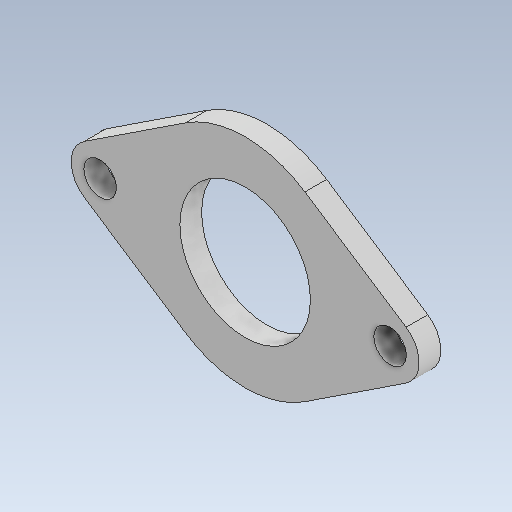
# Autodesk Inventor part: Peça27
Saved by Autodesk Inventor 2021 (Build 250183000, 183)
## iProperties
Created: 2021-07-21
Part Number: Peça27
Material: Genérico
Document SubType Name: Modeling
Designer: Giovanni
Density: 1 g/cm^3
Appearance: Padrão
Author: Giovanni
Autodesk Inventor part; units mm, degrees
ref_plane "YZ Plane" through (0, 0, 0) normal (1, 0, 0) x (0, 1, 0)
ref_plane "XZ Plane" through (0, 0, 0) normal (0, 1, 0) x (-1, 0, 0)
ref_plane "XY Plane" through (0, 0, 0) normal (0, 0, 1) x (1, 0, 0)
sketch "Esboço1" plane through (0, 0, 0) normal (0, 0, 1) x (1, 0, 0)
  arc A0 (-22.2, 3.3407) -> (-22.2, -3.3407) centre (-20, 0) ccw
  arc A1 (22.2, -3.3407) -> (22.2, 3.3407) centre (20, 0) ccw
  line L0 (-8.25, 12.5275) -> (-22.2, 3.3407)
  line L1 (-22.2, -3.3407) -> (-8.25, -12.5275)
  line L2 (8.25, -12.5275) -> (22.2, -3.3407)
  line L3 (22.2, 3.3407) -> (8.25, 12.5275)
  arc A2 (-8.25, -12.5275) -> (8.25, -12.5275) centre (0, 0) ccw
  arc A3 (8.25, 12.5275) -> (-8.25, 12.5275) centre (0, 0) ccw
  circle A4 centre (0, 0) radius 9
  circle A5 centre (20, 0) radius 2.25
  circle A6 centre (-20, 0) radius 2.25
  dimension "d1" = 8
  dimension "d2" = 20
  dimension "d3" = 20
  dimension "d4" = 18
  dimension "d5" = 4.5
  dimension "d6" = 15
  constraints: 8 end point, 8 point on circle, 8 tangent, 7 centre point, 4 coincident, 3 equal radius
  measures "d1" diameter of A0
  measures "d2" distance of point (0, 0) A0.centre
  measures "d3" distance of A1.centre point (0, 0)
  measures "d4" diameter of A4
  measures "d5" diameter of A5
  measures "d6" radius of A3
extrude "Extrusão1" add sketch "Esboço1" along normal blind 3
